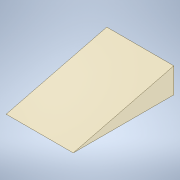
# Autodesk Inventor part: roof
Saved by Autodesk Inventor 2021.1 (Build 251245000, 245)
## iProperties
Created: 2020-03-27
Part Number: roof
Material: PET Plastic
Document SubType Name: Modeling
Designer: robst
Density: 1.541 g/cm^3
Appearance: Light Beige
Author: robst
Autodesk Inventor part; units mm, degrees
ref_plane "YZ Plane" through (0, 0, 0) normal (1, 0, 0) x (0, 1, 0)
ref_plane "XZ Plane" through (0, 0, 0) normal (0, 1, 0) x (-1, 0, 0)
ref_plane "XY Plane" through (0, 0, 0) normal (0, 0, 1) x (1, 0, 0)
sketch "Sketch1" plane through (0, 0, 0) normal (1, 0, 0) x (0, 1, 0)
  line L0 (0, 0) -> (914.4, 0)
  line L1 (914.4, 0) -> (0, 3657.6)
  line L2 (0, 3657.6) -> (0, 0)
  line L3 (914.4, 0) -> (2396.8282, -1624.8847)
  line L4 (2396.8282, -1624.8847) -> (914.4, -1624.8847)
  line L5 (914.4, -1624.8847) -> (914.4, 0)
  line L6 (0, 0) -> (0, -1624.8847)
  line L7 (0, -1624.8847) -> (914.4, -1624.8847)
  dimension "rise" = 914.4
  dimension "run" = 3657.6
  dimension "roofAngle" = 14.036
  constraints: 16 end point, 2 horizontal, 2 perpendicular, 2 vertical
  measures "rise" distance of L0.start L0.end
  measures "run" distance of L1.end L0.start
  measures "roofAngle" angle of L1 L2
extrude "Extrusion1" add sketch "Sketch1" along normal mid plane 2438.4 contours L2 L1 L0
body "Solid1"
